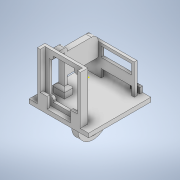
# Autodesk Inventor part: MOUSE SIP
Saved by Autodesk Inventor 2022 (Build 260153000, 153)
## iProperties
Created: 2024-03-04
Part Number: MOUSE SIP
Material: Generic
Document SubType Name: Modeling
Designer: admin
Density: 1 g/cm^3
Appearance: Default
Author: admin
Autodesk Inventor part; units mm, degrees
ref_plane "YZ Plane" through (0, 0, 0) normal (1, 0, 0) x (0, 1, 0)
ref_plane "XZ Plane" through (0, 0, 0) normal (0, 1, 0) x (-1, 0, 0)
ref_plane "XY Plane" through (0, 0, 0) normal (0, 0, 1) x (1, 0, 0)
sketch "Sketch1" plane through (0, 0, 0) normal (0, 1, 0) x (-1, 0, 0)
  line L0 (0, 0) -> (43, 0)
  line L1 (43, 0) -> (43, -45)
  line L2 (43, -45) -> (0, -45)
  line L3 (0, -45) -> (0, 0)
  dimension "d0" = 43
  dimension "d1" = 45
  constraints: 8 end point, 2 parallel, 1 horizontal, 1 perpendicular
  measures "d0" distance of L1.end L2.end
  measures "d1" distance between parallel lines of L2 L0
extrude "Extrusion1" add sketch "Sketch1" along normal blind 38
sketch "Sketch2" plane through (0, 38, 0) normal (0, 1, 0) x (1, 0, 0)
  point P0 (0, 0)
sketch "Sketch3" plane through (0, 38, 0) normal (0, 1, 0) x (1, 0, 0)
  line L0 (-43, 45) -> (-43, 0) projected
  line L1 (-43, 0) -> (-37, 0)
  line L2 (-37, 0) -> (-37, 5.5)
  line L3 (-37, 5.5) -> (-43, 5.5)
  line L4 (-43, 5.5) -> (-43, 0)
  line L5 (-43, 0) -> (0, 0) projected
  line L6 (0, 0) -> (-6, 0)
  line L7 (-6, 0) -> (-6, 5.5)
  line L8 (-6, 5.5) -> (0, 5.5)
  line L9 (0, 5.5) -> (0, 0)
  line L10 (-37, 0) -> (-30, 0)
  line L11 (-30, 0) -> (-30, 2)
  line L12 (-30, 2) -> (-37, 2)
  line L13 (-37, 2) -> (-37, 0)
  line L14 (-6, 0) -> (-13, 0)
  line L15 (-13, 0) -> (-13, 2)
  line L16 (-13, 2) -> (-6, 2)
  line L17 (-6, 2) -> (-6, 0)
  line L18 (-37, 2) -> (-35, 2)
  line L19 (-35, 2) -> (-35, 5.5)
  line L20 (-35, 5.5) -> (-37, 5.5)
  line L21 (-37, 5.5) -> (-37, 2)
  line L22 (-6, 2) -> (-8, 2)
  line L23 (-8, 2) -> (-8, 5.5)
  line L24 (-8, 5.5) -> (-6, 5.5)
  line L25 (-6, 5.5) -> (-6, 2)
  line L26 (-35, 2) -> (-8, 2)
  line L27 (-8, 2) -> (-8, 3.5)
  line L28 (-8, 3.5) -> (-35, 3.5)
  line L29 (-35, 3.5) -> (-35, 2)
  line L30 (-35, 2) -> (-37, 2)
  line L31 (-37, 2) -> (-37, 0)
  line L32 (-37, 0) -> (-35, 0)
  line L33 (-35, 0) -> (-35, 2)
  line L34 (-8, 2) -> (-6, 2)
  line L35 (-6, 2) -> (-6, 0)
  line L36 (-6, 0) -> (-8, 0)
  line L37 (-8, 0) -> (-8, 2)
  dimension "d4" = 6
  dimension "d5" = 5.5
  dimension "d6" = 6
  dimension "d7" = 5.5
  dimension "d8" = 7
  dimension "d9" = 2
  dimension "d10" = 7
  dimension "d11" = 2
  dimension "d12" = 2
  dimension "d13" = 2
  dimension "d14" = 1.5
  constraints: 72 end point, 18 parallel, 9 horizontal, 9 perpendicular, 2 point on line
  measures "d4" distance of L3.end L2.end
  measures "d5" distance of L2.end L1.end
  measures "d6" distance of L7.end L8.end
  measures "d7" distance of L6.end L7.end
  measures "d8" distance of L12.end L11.end
  measures "d9" distance of L11.end L10.end
  measures "d10" distance of L15.end L16.end
  measures "d11" distance of L14.end L15.end
  measures "d12" distance of L20.end L19.end
  measures "d13" distance of L23.end L24.end
  measures "d14" distance of L27.end L26.end
extrude "Extrusion2" cut sketch "Sketch3" against normal blind 35 contours L3 L2 L1 L0 | L19 L28 L23 L16 L26 L12 | L7 L8 L9 L5
extrude "Extrusion3" cut sketch "Sketch3" against normal blind 27 contours L33 L12 L11 L5 | L15 L16 L37 L5
extrude "Extrusion4" cut sketch "Sketch3" against normal blind 35 contours L11 L26 L15 L5
sketch "Sketch4" plane through (0, 38, 0) normal (0, 1, 0) x (1, 0, 0)
  line L0 (0, 45) -> (-43, 45) projected
  line L1 (-43, 45) -> (-41, 45)
  line L2 (-41, 45) -> (-41, 35)
  line L3 (-41, 35) -> (-43, 35)
  line L4 (-43, 35) -> (-43, 45)
  line L5 (-41, 45) -> (-34, 45)
  line L6 (-34, 45) -> (-34, 43)
  line L7 (-34, 43) -> (-41, 43)
  line L8 (-41, 43) -> (-41, 45)
  line L9 (-41, 43) -> (-6, 43)
  line L10 (-6, 43) -> (-6, 41)
  line L11 (-6, 41) -> (-41, 41)
  line L12 (-41, 41) -> (-41, 43)
  line L13 (-6, 43) -> (-13, 43)
  line L14 (-13, 43) -> (-13, 45)
  line L15 (-13, 45) -> (-6, 45)
  line L16 (-6, 45) -> (-6, 43)
  line L17 (-41, 41) -> (-6, 41)
  line L18 (-6, 41) -> (-6, 36)
  line L19 (-6, 36) -> (-41, 36)
  line L20 (-41, 36) -> (-41, 41)
  point P0 (0, 0)
  dimension "d21" = 2
  dimension "d22" = 10
  dimension "d23" = 7
  dimension "d24" = 2
  dimension "d25" = 35
  dimension "d26" = 2
  dimension "d27" = 7
  dimension "d28" = 35
  dimension "d29" = 5
  constraints: 40 end point, 10 parallel, 5 horizontal, 5 perpendicular, 1 point on line
  measures "d21" distance of L2.end L3.end
  measures "d22" distance of L1.end L2.end
  measures "d23" distance of L6.end L7.end
  measures "d24" distance of L5.end L6.end
  measures "d25" distance of L10.end L11.end
  measures "d26" distance of L9.end L10.end
  measures "d27" distance of L14.end L15.end
  measures "d28" distance of L18.end L19.end
  measures "d29" distance of L17.end L18.end
extrude "Extrusion5" cut sketch "Sketch4" against normal blind 35 contours L14 L9 L6 L0 | L10 L11 L2 L7 L9
extrude "Extrusion6" cut sketch "Sketch4" against normal blind 29 contours L16 L9 L14 L0 | L6 L7 L2 L0 | L2 L3 L4 L0
sketch "Sketch5" plane through (0, 38, 0) normal (0, 1, 0) x (1, 0, 0)
  line L0 (-43, 5.5) -> (-37, 5.5) projected
  line L1 (-6, 0) -> (-6, 5.5) projected
  line L2 (-37, 5.5) -> (-6, 5.5)
  line L3 (-6, 5.5) -> (-6, 3.5)
  line L4 (-6, 3.5) -> (-37, 3.5)
  line L5 (-37, 3.5) -> (-37, 5.5)
  line L6 (-43, 35) -> (-43, 5.5) projected
  line L7 (0, 5.5) -> (-43, 5.5)
  line L8 (-43, 5.5) -> (-43, 35)
  line L9 (-43, 35) -> (0, 35)
  line L10 (0, 35) -> (0, 5.5)
  line L11 (-6, 41) -> (-41, 41) projected
  line L12 (0, 35) -> (-41, 35)
  line L13 (-41, 35) -> (-41, 41)
  line L14 (-41, 41) -> (0, 41)
  line L15 (0, 41) -> (0, 35)
  line L16 (-6, 45) -> (-6, 41) projected
  line L17 (-6, 45) -> (0, 45)
  line L18 (0, 45) -> (0, 41)
  line L19 (0, 41) -> (-6, 41)
  line L20 (-6, 41) -> (-6, 45)
  point P0 (0, 0)
  dimension "d34" = 2
  constraints: 32 end point, 8 parallel, 4 horizontal, 4 perpendicular, 1 point on line
  measures "d34" distance of L2.end L3.end
extrude "Extrusion7" cut sketch "Sketch5" against normal blind 5 contours L6 L9 L10 L7 L2 L0 | L13 L11 L14 L15 L9
extrude "Extrusion8" cut sketch "Sketch5" against normal blind 35 contours L14 L16 L17 L18
sketch "Sketch6" plane through (0, 33, 0) normal (0, 1, 0) x (1, 0, 0)
  line L0 (0, 41) -> (-41, 41) projected
  line L1 (-41, 41) -> (-6, 41)
  line L2 (-6, 41) -> (-6, 39)
  line L3 (-6, 39) -> (-41, 39)
  line L4 (-41, 39) -> (-41, 41)
  line L5 (-6, 5.5) -> (-37, 5.5) projected
  line L6 (-37, 5.5) -> (-36, 5.5)
  line L7 (-36, 5.5) -> (-36, 6.5)
  line L8 (-36, 6.5) -> (-37, 6.5)
  line L9 (-37, 6.5) -> (-37, 5.5)
  line L10 (-36, 5.5) -> (-32, 5.5)
  line L11 (-32, 5.5) -> (-32, 39)
  line L12 (-32, 39) -> (-36, 39)
  line L13 (-36, 39) -> (-36, 5.5)
  line L14 (-43, 5.5) -> (-43, 35) projected
  line L15 (-43, 35) -> (-36, 35)
  line L16 (-36, 35) -> (-36, 5.5)
  line L17 (-36, 5.5) -> (-43, 5.5)
  line L18 (-43, 5.5) -> (-43, 35)
  line L19 (-41, 39) -> (-36, 39)
  line L20 (-36, 39) -> (-36, 35)
  line L21 (-36, 35) -> (-41, 35)
  line L22 (-41, 35) -> (-41, 39)
  line L23 (0, 41) -> (0, 5.5) projected
  line L24 (0, 5.5) -> (-32, 5.5)
  line L25 (-32, 5.5) -> (-32, 39)
  line L26 (-32, 39) -> (0, 39)
  line L27 (0, 39) -> (0, 5.5)
  line L28 (0, 39) -> (-6, 39)
  line L29 (-6, 39) -> (-6, 41)
  line L30 (-6, 41) -> (0, 41)
  line L31 (0, 41) -> (0, 39)
  point P0 (0, 0)
  point P1 (-32, 5.5)
  point P2 (-6, 41)
  point P3 (0, 39)
  dimension "d39" = 35
  dimension "d40" = 2
  dimension "d41" = 1
  dimension "d42" = 1
  dimension "d43" = 4
  constraints: 56 end point, 14 parallel, 7 horizontal, 7 perpendicular, 1 point on line
  measures "d39" distance of L2.end L3.end
  measures "d40" distance of L1.end L2.end
  measures "d41" distance of L8.end L7.end
  measures "d42" distance of L7.end L6.end
  measures "d43" distance of L12.end L11.end
extrude "Extrusion9" cut sketch "Sketch6" against normal blind 30 contours L23 L26 L2 L0 | L23 L24 L5 L11 L3 L26 | L3 L13 L15 L22 | L15 L13 L8 L9 L17 L14 | L5 L9 L8 L7
sketch "Sketch9" plane through (0, 9, 0) normal (0, 1, 0) x (1, 0, 0)
  line L0 (-41, 39) -> (-41, 35) projected
  line L1 (-43, 35) -> (-43, 45) projected
  line L2 (-41, 39) -> (-43, 39)
  line L3 (-43, 39) -> (-43, 35)
  line L4 (-43, 35) -> (-41, 35)
  line L5 (-41, 35) -> (-41, 39)
  point P0 (0, 0)
  constraints: 8 end point, 2 parallel, 1 horizontal, 1 perpendicular
extrude "Extrusion11" cut sketch "Sketch9" against normal blind 6
sketch "Sketch10" plane through (-36, 33, -39) normal (-1, 0, 0) x (0, 0, 1)
  line L0 (33.5, 0) -> (33.5, -30) projected
  line L1 (33.5, -30) -> (26.5, -30)
  line L2 (26.5, -30) -> (26.5, -3)
  line L3 (26.5, -3) -> (33.5, -3)
  line L4 (33.5, -3) -> (33.5, -30)
  line L5 (26.5, -30) -> (24.5, -30)
  line L6 (24.5, -30) -> (24.5, -24)
  line L7 (24.5, -24) -> (26.5, -24)
  line L8 (26.5, -24) -> (26.5, -30)
  line L9 (33.5, 0) -> (0, 0) projected
  line L10 (24.5, -30) -> (22.5, -30)
  line L11 (22.5, -30) -> (22.5, 0)
  line L12 (22.5, 0) -> (24.5, 0)
  line L13 (24.5, 0) -> (24.5, -30)
  line L14 (22.5, -30) -> (20.5, -30)
  line L15 (20.5, -30) -> (20.5, -24)
  line L16 (20.5, -24) -> (22.5, -24)
  line L17 (22.5, -24) -> (22.5, -30)
  line L18 (33.5, -30) -> (0, -30) projected
  line L19 (0, -30) -> (20.5, -30)
  line L20 (20.5, -30) -> (20.5, -24)
  line L21 (20.5, -24) -> (0, -24)
  line L22 (0, -24) -> (0, -30)
  line L23 (0, -24) -> (0, 0) projected
  line L24 (0, -24) -> (22.5, -24)
  line L25 (22.5, -24) -> (22.5, -18)
  line L26 (22.5, -18) -> (0, -18)
  line L27 (0, -18) -> (0, -24)
  line L28 (0, -18) -> (22.5, -18)
  line L29 (22.5, -18) -> (22.5, -3)
  line L30 (22.5, -3) -> (0, -3)
  line L31 (0, -3) -> (0, -18)
  line L32 (0, -3) -> (22.5, -3)
  line L33 (22.5, -3) -> (22.5, 0)
  line L34 (22.5, 0) -> (0, 0)
  line L35 (0, 0) -> (0, -3)
  line L36 (24.5, -24) -> (26.5, -24)
  line L37 (26.5, -24) -> (26.5, -3)
  line L38 (26.5, -3) -> (24.5, -3)
  line L39 (24.5, -3) -> (24.5, -24)
  line L40 (22.5, -30) -> (24.5, -30)
  line L41 (24.5, -30) -> (24.5, -24)
  line L42 (24.5, -24) -> (22.5, -24)
  line L43 (22.5, -24) -> (22.5, -30)
  point P0 (39, -33)
  point P1 (0, -18)
  point P2 (33.5, -3)
  dimension "d59" = 7
  dimension "d60" = 27
  dimension "d61" = 2
  dimension "d62" = 6
  dimension "d63" = 2
  dimension "d64" = 2
  dimension "d65" = 6
  constraints: 80 end point, 20 parallel, 10 horizontal, 10 perpendicular, 3 point on line
  measures "d59" distance of L2.end L3.end
  measures "d60" distance of L1.end L2.end
  measures "d61" distance of L6.end L7.end
  measures "d62" distance of L5.end L6.end
  measures "d63" distance of L11.end L12.end
  measures "d64" distance of L15.end L16.end
  measures "d65" distance of L25.end L24.end
extrude "Extrusion12" cut sketch "Sketch10" against normal blind 6 contours L0 L1 L2 L3 | L2 L7 L13 L38 | L11 L30 L23 L9 | L11 L16 L21 L23 L26 | L15 L18 L22 L21
extrude "Extrusion13" add sketch "Sketch10" along normal blind 2 and the other way blind 6 contours L5 L6 L7 L2 | L6 L10 L11 L42 | L11 L14 L15 L16
sketch "Sketch12" plane through (-35, 38, -3.5) normal (0, 0, 1) x (1, 0, 0)
  line L0 (0, -35) -> (6, -35)
  line L1 (6, -35) -> (6, -29)
  line L2 (6, -29) -> (0, -29)
  line L3 (0, -29) -> (0, -35)
  line L4 (0, 0) -> (0, -35) projected
  line L5 (0, 0) -> (6, 0)
  line L6 (6, 0) -> (6, -6)
  line L7 (6, -6) -> (0, -6)
  line L8 (0, -6) -> (0, 0)
  line L9 (0, -35) -> (27, -35) projected
  line L10 (27, -35) -> (21, -35)
  line L11 (21, -35) -> (21, -29)
  line L12 (21, -29) -> (27, -29)
  line L13 (27, -29) -> (27, -35)
  line L14 (0, 0) -> (27, 0) projected
  line L15 (27, 0) -> (21, 0)
  line L16 (21, 0) -> (21, -6)
  line L17 (21, -6) -> (27, -6)
  line L18 (27, -6) -> (27, 0)
  line L19 (6, -29) -> (0, -29)
  line L20 (0, -29) -> (0, -6)
  line L21 (0, -6) -> (6, -6)
  line L22 (6, -6) -> (6, -29)
  line L23 (6, -6) -> (21, -6)
  line L24 (21, -6) -> (21, 0)
  line L25 (21, 0) -> (6, 0)
  line L26 (6, 0) -> (6, -6)
  line L27 (21, -29) -> (27, -29)
  line L28 (27, -29) -> (27, -6)
  line L29 (27, -6) -> (21, -6)
  line L30 (21, -6) -> (21, -29)
  line L31 (6, 0) -> (21, 0)
  line L32 (21, 0) -> (21, -3)
  line L33 (21, -3) -> (6, -3)
  line L34 (6, -3) -> (6, 0)
  line L35 (3, -5) -> (3, -8) projected
  line L36 (0, -29) -> (3, -29)
  line L37 (3, -29) -> (3, -6)
  line L38 (3, -6) -> (0, -6)
  line L39 (0, -6) -> (0, -29)
  line L40 (27, -29) -> (24, -29)
  line L41 (24, -29) -> (24, -6)
  line L42 (24, -6) -> (27, -6)
  line L43 (27, -6) -> (27, -29)
  line L44 (6, -35) -> (21, -35)
  line L45 (21, -35) -> (21, -32)
  line L46 (21, -32) -> (6, -32)
  line L47 (6, -32) -> (6, -35)
  point P0 (35, -38)
  point P1 (21, -3)
  point P2 (6, -3)
  dimension "d79" = 6
  dimension "d80" = 6
  dimension "d81" = 6
  dimension "d82" = 6
  dimension "d83" = 6
  dimension "d84" = 6
  dimension "d85" = 6
  dimension "d86" = 6
  dimension "d87" = 3
  dimension "d88" = 3
  constraints: 88 end point, 22 parallel, 11 horizontal, 11 perpendicular, 4 midpoint, 1 point on line
  measures "d79" distance of L2.end L1.end
  measures "d80" distance of L1.end L0.end
  measures "d81" distance of L6.end L7.end
  measures "d82" distance of L5.end L6.end
  measures "d83" distance of L11.end L12.end
  measures "d84" distance of L10.end L11.end
  measures "d85" distance of L17.end L16.end
  measures "d86" distance of L16.end L15.end
  measures "d87" distance of L31.end L32.end
  measures "d88" distance of L45.end L44.end
extrude "Extrusion15" cut sketch "Sketch12" against normal blind 2 contours L1 L22 L23 L30 L11 L46 | L37 L35 L7 L22 L2 | L6 L33 L16 L23 | L30 L17 L41 L12
fillet "Fillet2" radius 2 9 edges at (-34, 33, -16.5) (-14, 32, -4.5) (-14, 9, -4.5) (-34, 9, -12.5) (-34, 9, -18.5) (-38, 9, -15.5) (-29, 32, -4.5) (-29, 9, -4.5) (-30, 9, -15.5)
sketch "Sketch13" plane through (0, 33, 0) normal (0, 1, 0) x (1, 0, 0)
  line L0 (-41, 41) -> (-6, 41) projected
  line L1 (-41, 39) -> (-6, 39)
  line L2 (-6, 39) -> (-6, 41)
  line L3 (-6, 41) -> (-41, 41)
  line L4 (-41, 41) -> (-41, 39)
  point P0 (0, 0)
  constraints: 8 end point, 2 parallel, 1 horizontal, 1 perpendicular
extrude "Extrusion16" cut sketch "Sketch13" against normal blind 8
fillet "Fillet3" radius 5 1 edges at (-34, 30, -39)
sketch "Sketch14" plane through (-43, 3, -39) normal (0, 0, 1) x (1, 0, 0)
  line L0 (37, 22) -> (37, 0) projected
  line L1 (37, 0) -> (35, 0)
  line L2 (35, 0) -> (35, 6)
  line L3 (35, 6) -> (37, 6)
  line L4 (37, 6) -> (37, 0)
  line L5 (11, 22) -> (11, 12) projected
  line L6 (37, 6) -> (11, 6)
  line L7 (11, 6) -> (11, 13)
  line L8 (11, 13) -> (37, 13)
  line L9 (37, 13) -> (37, 6)
  line L10 (37, 0) -> (2, 0) projected
  line L11 (11, 6) -> (13, 6)
  line L12 (13, 6) -> (13, 0)
  line L13 (13, 0) -> (11, 0)
  line L14 (11, 0) -> (11, 6)
  line L15 (37, 22) -> (11, 22) projected
  line L16 (11, 13) -> (13, 13)
  line L17 (13, 13) -> (13, 22)
  line L18 (13, 22) -> (11, 22)
  line L19 (11, 22) -> (11, 13)
  line L20 (37, 13) -> (35, 13)
  line L21 (35, 13) -> (35, 22)
  line L22 (35, 22) -> (37, 22)
  line L23 (37, 22) -> (37, 13)
  line L24 (13, 22) -> (35, 22)
  line L25 (35, 22) -> (35, 20)
  line L26 (35, 20) -> (13, 20)
  line L27 (13, 20) -> (13, 22)
  line L28 (13, 20) -> (35, 20)
  line L29 (35, 20) -> (35, 13)
  line L30 (35, 13) -> (13, 13)
  line L31 (13, 13) -> (13, 20)
  point P0 (43, -3)
  point P1 (13, 6)
  point P2 (13, 13)
  dimension "d96" = 2
  dimension "d97" = 6
  dimension "d98" = 7
  dimension "d99" = 2
  dimension "d100" = 2
  dimension "d101" = 2
  dimension "d102" = 2
  constraints: 56 end point, 14 parallel, 7 horizontal, 7 perpendicular, 5 point on line
  measures "d96" distance of L2.end L3.end
  measures "d97" distance of L1.end L2.end
  measures "d98" distance of L6.end L7.end
  measures "d99" distance of L12.end L13.end
  measures "d100" distance of L18.end L17.end
  measures "d101" distance of L21.end L22.end
  measures "d102" distance of L24.end L25.end
extrude "Extrusion17" cut sketch "Sketch14" against normal blind 2 contours L8 L17 L26 L21 | L2 L10 L12 L6
sketch "Sketch15" plane through (0, 0, 0) normal (0, -1, 0) x (1, 0, 0)
  line L0 (0, 0) -> (-19.25, 0)
  line L1 (-19.25, 0) -> (-19.25, -45)
  line L2 (-19.25, -45) -> (0, -45)
  line L3 (0, -45) -> (0, 0)
  line L4 (-34, -45) -> (-13, -45) projected
  line L5 (-19.25, 0) -> (-23.75, 0)
  line L6 (-23.75, 0) -> (-23.75, -45)
  line L7 (-23.75, -45) -> (-19.25, -45)
  line L8 (-19.25, -45) -> (-19.25, 0)
  line L9 (-23.75, 0) -> (-19.25, 0)
  line L10 (-19.25, 0) -> (-19.25, -11.5)
  line L11 (-19.25, -11.5) -> (-23.75, -11.5)
  line L12 (-23.75, -11.5) -> (-23.75, 0)
  line L13 (-23.75, -11.5) -> (-19.25, -11.5)
  line L14 (-19.25, -11.5) -> (-19.25, -33.5)
  line L15 (-19.25, -33.5) -> (-23.75, -33.5)
  line L16 (-23.75, -33.5) -> (-23.75, -11.5)
  dimension "d105" = 19.25
  dimension "d106" = 4.5
  dimension "d119" = 11.5
  dimension "d120" = 22
  constraints: 32 end point, 8 parallel, 4 horizontal, 4 perpendicular, 3 point on line
  measures "d105" distance of L2.end L1.end
  measures "d106" distance of L7.end L6.end
  measures "d119" distance of L9.end L10.end
  measures "d120" distance of L13.end L14.end
extrude "Extrusion18" add sketch "Sketch15" along normal blind 22 contours L1 L15 L6 L11
sketch "Sketch16" plane through (-19.25, 0, 0) normal (1, 0, 0) x (0, 0, -1)
  line L0 (11.5, -22) -> (33.5, -22) projected
  circle A0 centre (22.5, -11) radius 3.5
  circle A1 centre (22.5, -11) radius 8
  line L1 (45, 0) -> (0, 0) projected
  line L2 (0, 0) -> (22.5, 0)
  line L3 (22.5, 0) -> (22.5, -11)
  line L4 (22.5, -11) -> (0, -11)
  line L5 (0, -11) -> (0, 0)
  point P0 (0, -25)
  point P1 (45, -25)
  dimension "d111" = 7
  dimension "d112" = 16
  dimension "d124" = 11
  constraints: 8 end point, 2 centre point, 2 coincident, 2 parallel, 1 horizontal, 1 perpendicular, 1 other
  measures "d111" diameter of A0
  measures "d112" diameter of A1
  measures "d124" distance of L2.end L3.end
extrude "Extrusion19" cut sketch "Sketch16" against normal blind 25 contours A0 L4 L3 | L3 L4 A0
extrude "Extrusion20" add sketch "Sketch16" along normal blind 0.5 and the other way blind 5 contours A0 L3 A1 L4 | A0 L4 A1 L3
fillet "Face Fillet1" radius 11.5 1 edges at (-21.5, 0, -11.5)
fillet "Face Fillet2" radius 11.5 1 edges at (-21.5, 0, -33.5)
fillet "Fillet4" radius 11 2 edges at (-21.5, -22, -33.5) (-21.5, -22, -11.5)
sketch "Sketch17" plane through (0, 9, 0) normal (0, 1, 0) x (1, 0, 0)
  line L0 (-6, 43) -> (-6, 45) projected
  line L1 (-6, 43) -> (-13, 43) projected
  line L2 (-6, 45) -> (-13, 45)
  line L3 (-13, 45) -> (-13, 43)
  line L4 (-13, 43) -> (-6, 43)
  line L5 (-6, 43) -> (-6, 45)
  line L6 (-43, 45) -> (-34, 45) projected
  line L7 (-43, 39) -> (-43, 45) projected
  line L8 (-34, 45) -> (-43, 45)
  line L9 (-43, 45) -> (-43, 43)
  line L10 (-43, 43) -> (-34, 43)
  line L11 (-34, 43) -> (-34, 45)
  line L12 (-41, 41) -> (-41, 39) projected
  line L13 (-43, 43) -> (-41, 43)
  line L14 (-41, 43) -> (-41, 39)
  line L15 (-41, 39) -> (-43, 39)
  line L16 (-43, 39) -> (-43, 43)
  point P0 (0, 0)
  constraints: 24 end point, 6 parallel, 3 horizontal, 3 perpendicular, 2 point on line
extrude "Extrusion21" cut sketch "Sketch17" against normal blind 2
body "Solid1"
